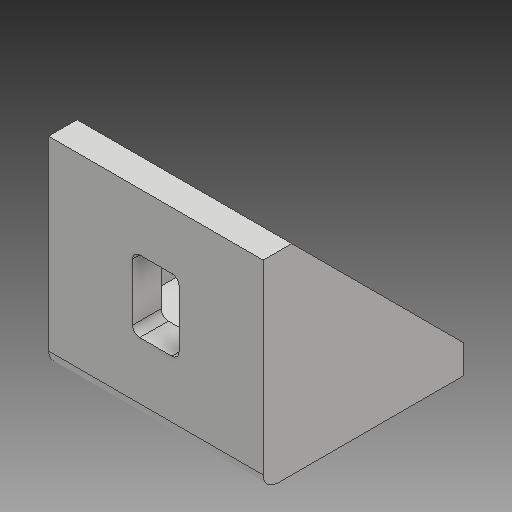
# Autodesk Inventor part: item_winkel
Saved by Autodesk Inventor 2018 (Build 220112000, 112)
## iProperties
Created: 2020-04-13
Part Number: item_winkel
Material: Generisch
Document SubType Name: Modeling
Designer: wepet
Density: 1 g/cm^3
Appearance: Vorgabe
Description: Eckwinkel für Aluprofil 30x30
Mass: 0.00694239 g
Surface Area: 0.478649 cm^2
Volume: 0.00694239 cm^3
Author: wepet
Autodesk Inventor part; units mm, degrees
ref_plane "YZ Plane" through (0, 0, 0) normal (1, 0, 0) x (0, 1, 0)
ref_plane "XZ Plane" through (0, 0, 0) normal (0, 1, 0) x (-1, 0, 0)
ref_plane "XY Plane" through (0, 0, 0) normal (0, 0, 1) x (1, 0, 0)
sketch "Skizze2" plane through (0, 0, 0) normal (1, 0, 0) x (0, 1, 0)
  line L0 (0, 0) -> (2.8, 0) construction
  line L1 (2.8, 0) -> (2.8, 2.8) construction
  line L2 (2.8, 2.8) -> (0, 2.8) construction
  line L3 (0, 2.8) -> (0, 0) construction
  line L4 (0.4, 2.8) -> (0.4, 0) construction
  line L5 (0, 0.4) -> (2.8, 0.4) construction
  line L6 (0, 0.2) -> (0, 2.8)
  line L7 (0.4, 2.8) -> (0.4, 0.8)
  line L8 (2.8, 0.4) -> (0.8, 0.4)
  line L9 (0, 2.8) -> (0.4, 2.8)
  line L10 (2.8, 0) -> (2.8, 0.4)
  line L11 (2.8, 0) -> (0.2, 0)
  arc A0 (0, 0.2) -> (0.2, 0) centre (0.2, 0.2) ccw
  arc A1 (0.4, 0.8) -> (0.8, 0.4) centre (0.8, 0.8) ccw
  point P0 (0.4, 0.4)
  dimension "d0" = 2.8
  dimension "d1" = 2.8
  dimension "d2" = 0.4
  dimension "d3" = 0.4
  dimension "d4" = 0.2
  dimension "d5" = 0.4
  constraints: 24 end point, 10 point on line, 4 collinear, 4 perpendicular, 4 point on circle, 4 tangent, 2 centre point, 2 parallel, 1 horizontal
  measures "d0" distance of L2.end L1.end
  measures "d1" distance of L1.end L0.end
  measures "d2" distance between parallel lines of L3 L4
  measures "d3" distance between parallel lines of L0 L5
  measures "d4" radius of A0
  measures "d5" radius of A1
extrude "Extrusion1" add sketch "Skizze2" along normal blind 2.6
sketch "Skizze3" plane through (2.6, 0, 0) normal (1, 0, 0) x (0, 0, -1)
  line L0 (0, 2.8) -> (-0.4, 2.8) projected
  line L1 (-0.4, 2.8) -> (-0.4, 0.8) construction
  arc A0 (-0.8, 0.4) -> (-0.4, 0.8) centre (-0.8, 0.8) ccw construction
  line L2 (-0.8, 0.4) -> (-2.8, 0.4) construction
  line L3 (-2.8, 0.4) -> (-2.8, 0) projected
  line L4 (-2.8, 0) -> (-0.2, 0) projected
  arc A1 (-0.2, 0) -> (0, 0.2) centre (-0.2, 0.2) ccw projected
  line L5 (0, 0.2) -> (0, 2.8) projected
  line L6 (-2.8, 0.4) -> (-2.8, 0) projected
  line L7 (-2.8, 0.4) -> (-0.4, 2.8)
  point P0 (0, 0)
  constraints: 2 end point
extrude "Extrusion2" add sketch "Skizze3" along normal blind 0.2
sketch "Skizze4" plane through (0, 0, 0) normal (-1, 0, 0) x (0, 0, 1)
  line L0 (0, 2.8) -> (0.4, 2.8) projected
  line L1 (0, 0.2) -> (0, 2.8) projected
  arc A0 (0, 0.2) -> (0.2, 0) centre (0.2, 0.2) ccw projected
  line L2 (2.8, 0) -> (0.2, 0) projected
  line L3 (2.8, 0.4) -> (2.8, 0) projected
  line L4 (0.8, 0.4) -> (2.8, 0.4) construction
  arc A1 (0.4, 0.8) -> (0.8, 0.4) centre (0.8, 0.8) ccw construction
  line L5 (0.4, 2.8) -> (0.4, 0.8) construction
  line L6 (0, 2.8) -> (0.4, 2.8) projected
  line L7 (2.8, 0.4) -> (2.8, 0) projected
  line L8 (0.4, 2.8) -> (2.8, 0.4)
  point P0 (0, 0)
  constraints: 2 end point
extrude "Extrusion3" add sketch "Skizze4" along normal blind 0.2
sketch "Skizze5" plane through (2.8, 0, 0.2) normal (0, -1, 0) x (1, 0, 0)
  line L0 (-3, 0) -> (0, 0) construction
  line L1 (0, 2.6) -> (0, 0) construction
  line L2 (-3, 2.6) -> (0, 2.6) construction
  line L3 (-3, 0) -> (-3, 2.6) construction
  line L4 (-1.5, 2.6) -> (-1.5, 0) construction
  line L5 (-3, 0) -> (0, 0) projected
  line L6 (-3, 0) -> (-3, 2.6) construction
  line L7 (-3, 1.3) -> (0, 1.3) construction
  line L8 (-1.725, 1.8) -> (-1.275, 1.8)
  line L9 (-1.175, 1.7) -> (-1.175, 0.9)
  line L10 (-1.275, 0.8) -> (-1.725, 0.8)
  line L11 (-1.825, 0.9) -> (-1.825, 1.7)
  arc A0 (-1.725, 1.8) -> (-1.825, 1.7) centre (-1.725, 1.7) ccw
  arc A1 (-1.275, 0.8) -> (-1.175, 0.9) centre (-1.275, 0.9) ccw
  arc A2 (-1.825, 0.9) -> (-1.725, 0.8) centre (-1.725, 0.9) ccw
  arc A3 (-1.175, 1.7) -> (-1.275, 1.8) centre (-1.275, 1.7) ccw
  point P0 (-2.8, -0.2)
  point P1 (-1.825, 1.8)
  point P2 (-1.175, 1.8)
  point P3 (-1.825, 0.8)
  point P4 (-1.825, 1.3)
  point P5 (-1.5, 1.8)
  dimension "d12" = 0.65
  dimension "d13" = 1
  dimension "d14" = 0.1
  constraints: 12 end point, 8 point on circle, 8 point on line, 8 tangent, 6 midpoint, 4 centre point, 3 equal radius, 2 parallel, 1 horizontal, 1 perpendicular
  measures "d12" distance of point (-1.825, 1.8) point (-1.175, 1.8)
  measures "d13" distance of point (-1.825, 0.8) point (-1.825, 1.8)
  measures "d14" radius of A0
extrude "Extrusion4" cut sketch "Skizze5" against normal blind 0.4
sketch "Skizze6" plane through (2.8, 0.2, 0) normal (0, 0, -1) x (-1, 0, 0)
  line L0 (0, 2.6) -> (3, 2.6) construction
  line L1 (0, 0) -> (0, 2.6) construction
  line L2 (3, 0) -> (0, 0) construction
  line L3 (3, 2.6) -> (3, 0) construction
  line L4 (3, 0) -> (0, 0) construction
  line L5 (1.5, 0) -> (1.5, 2.6) construction
  line L6 (2.8, 2.6) -> (0.2, 2.6) construction
  line L7 (3, 1.3) -> (0, 1.3) construction
  line L8 (1.725, 0.8) -> (1.275, 0.8)
  line L9 (1.175, 0.9) -> (1.175, 1.7)
  line L10 (1.275, 1.8) -> (1.725, 1.8)
  line L11 (1.825, 1.7) -> (1.825, 0.9)
  arc A0 (1.175, 0.9) -> (1.275, 0.8) centre (1.275, 0.9) ccw
  arc A1 (1.275, 1.8) -> (1.175, 1.7) centre (1.275, 1.7) ccw
  arc A2 (1.825, 1.7) -> (1.725, 1.8) centre (1.725, 1.7) ccw
  arc A3 (1.725, 0.8) -> (1.825, 0.9) centre (1.725, 0.9) ccw
  point P0 (2.8, -0.2)
  point P1 (1.825, 0.8)
  point P2 (1.175, 0.8)
  point P3 (1.825, 1.8)
  point P4 (1.5, 0.8)
  point P5 (1.175, 1.3)
  dimension "d17" = 1
  dimension "d18" = 0.65
  dimension "d19" = 0.1
  constraints: 12 end point, 8 point on circle, 8 point on line, 8 tangent, 6 midpoint, 4 centre point, 3 equal radius, 2 parallel, 1 horizontal, 1 perpendicular
  measures "d17" distance of point (1.825, 1.8) point (1.825, 0.8)
  measures "d18" distance of point (1.825, 0.8) point (1.175, 0.8)
  measures "d19" radius of A0
extrude "Extrusion5" cut sketch "Skizze6" against normal blind 0.4
